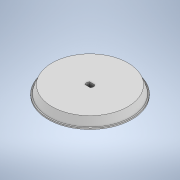
# Autodesk Inventor part: Wheel
Saved by Autodesk Inventor 2022 (Build 260153000, 153)
## iProperties
Created: 2022-03-28
Part Number: Wheel
Material: Generic
Document SubType Name: Modeling
Designer: Trushika
Density: 1 g/cm^3
Appearance: Default
Author: Trushika
Autodesk Inventor part; units mm, degrees
ref_plane "YZ Plane" through (0, 0, 0) normal (1, 0, 0) x (0, 1, 0)
ref_plane "XZ Plane" through (0, 0, 0) normal (0, 1, 0) x (-1, 0, 0)
ref_plane "XY Plane" through (0, 0, 0) normal (0, 0, 1) x (1, 0, 0)
sketch "Sketch1" plane through (0, 0, 0) normal (1, 0, 0) x (0, 1, 0)
  line L0 (0, 0) -> (0, -32.5)
  line L1 (0, -32.5) -> (1, -32.5)
  line L2 (1, -32.5) -> (1, -31.5)
  line L3 (1, -31.5) -> (7, -29.3162)
  line L4 (1, -31.5) -> (7.3851, -31.5) construction
  line L5 (7, -29.3162) -> (7, 0)
  line L6 (7, 0) -> (0, 0)
  dimension "d0" = 32.5
  dimension "d2" = 1
  dimension "d3" = 20
  dimension "d5" = 7
  dimension "d6" = 1
  constraints: 14 end point, 3 perpendicular, 2 vertical, 1 equal length, 1 horizontal
  measures "d0" distance of L0.start L0.end
  measures "d2" distance of L1.end L2.end
  measures "d3" angle of L4 L3
  measures "d5" distance between parallel lines of L0 L5
  measures "d6" distance of L0.end L1.end
revolve "Revolution1" add sketch "Sketch1" angle 360 about axis through (0, 7, 0) along (0, -1, 0)
sketch "Sketch2" plane through (0, 7, 0) normal (0, 1, 0) x (1, 0, 0)
  line L0 (2.0347, 1.85) -> (-2.0347, 1.85)
  line L1 (2.0347, -1.85) -> (-2.0347, -1.85)
  arc A0 (2.0347, -1.85) -> (2.0347, 1.85) centre (0, 0) ccw
  arc A1 (-2.0347, 1.85) -> (-2.0347, -1.85) centre (0, 0) ccw
  dimension "d9" = 4.0694
  dimension "d10" = 3.7
  constraints: 4 end point, 4 point on circle, 2 centre point, 1 coincident, 1 horizontal
  measures "d9" distance of L0.start L0.end
  measures "d10" distance of L0.start L1.start
extrude "Extrusion1" cut sketch "Sketch2" against normal through all
body "Solid1"
